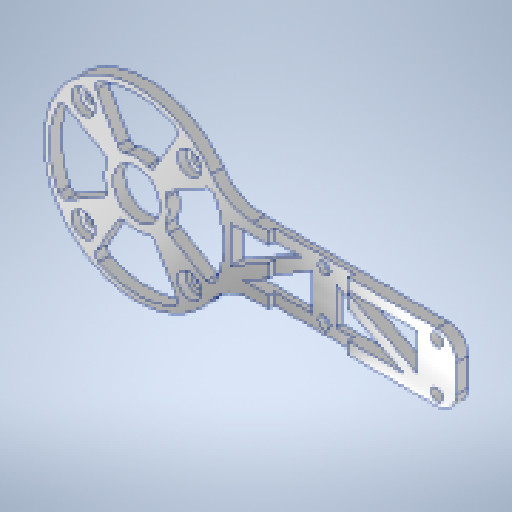
# Autodesk Inventor part: link2plate4
Saved by Autodesk Inventor 2024 (Build 280153000, 153)
## iProperties
Created: 2025-02-10
Part Number: link2plate4
Material: アルミニウム 6061
Document SubType Name: Modeling
Designer: tanoue_kota
Mass: 10.4195 g
Surface Area: 51.6889 cm^2
Volume: 3.85907 cm^3
Density: 2.7 g/cm^3
Appearance: アルミニウム - フラット
Author: tanoue_kota
Autodesk Inventor part; units mm, degrees
ref_plane "YZ Plane" through (0, 0, 0) normal (1, 0, 0) x (0, 1, 0)
ref_plane "XZ Plane" through (0, 0, 0) normal (0, 1, 0) x (-1, 0, 0)
ref_plane "XY Plane" through (0, 0, 0) normal (0, 0, 1) x (1, 0, 0)
sketch "スケッチ1" plane through (0, 0, 0) normal (0, 0, 1) x (1, 0, 0)
  line L0 (0, 0) -> (-81, 0)
  line L1 (-81, 0) -> (-81, 17)
  line L2 (-81, 17) -> (0, 17)
  line L3 (0, 17) -> (0, 0)
  line L4 (-81, 8.5) -> (0, 8.5)
  circle A0 centre (-81, 8.5) radius 23.5
  point P0 (-59.0911, 17)
  point P1 (-59.0911, 0)
  dimension "d0" = 17
  dimension "d28" = 47
  dimension "d29" = 81
  constraints: 10 end point, 2 midpoint, 2 parallel, 1 centre point, 1 coincident, 1 horizontal, 1 perpendicular
  measures "d0" distance of L2.end L0.start
  measures "d28" diameter of A0
  measures "d29" distance between parallel lines of L3 L1
extrude "押し出し1" add sketch "スケッチ1" along normal blind 3
sketch "スケッチ2" plane through (0, 0, 3) normal (0, 0, 1) x (1, 0, 0)
  line L0 (0, 0) -> (0, 17) projected
  line L1 (0, 8.5) -> (-59.0911, 8.5)
  line L2 (0, 17) -> (-59.0911, 17) projected
  line L3 (-5, 17) -> (-5, 0)
  line L4 (-35, 17) -> (-35, 0)
  line L5 (-59.0911, 0) -> (0, 0) projected
  arc A0 (-59.0911, 17) -> (-59.0911, 0) centre (-81, 8.5) ccw projected
  line L6 (-59.0911, 17) -> (-59.0911, 0)
  point P0 (-5, 14.5)
  point P1 (-35, 14.5)
  point P2 (-5, 2.5)
  point P3 (-35, 2.5)
  dimension "d4" = 5
  dimension "d5" = 30
  dimension "d6" = 6
  dimension "d7" = 6
  constraints: 8 end point, 5 point on line, 3 vertical, 2 midpoint, 2 symmetric about line, 1 parallel
  measures "d4" distance between parallel lines of L0 L3
  measures "d5" distance between parallel lines of L3 L4
  measures "d6" distance from line of L1 point (-5, 14.5)
  measures "d7" distance from line of L1 point (-35, 14.5)
hole "穴1" at (-5, 14.5, 3) at (-35, 14.5, 3) at (-35, 2.5, 3) at (-5, 2.5, 3) direction (0, 0, -1) diameter 3.1 depth 20 tip angle 118
sketch "スケッチ5" plane through (0, 0, 3) normal (0, 0, 1) x (1, 0, 0)
  arc A0 (-59.0911, 17) -> (-59.0911, 0) centre (-81, 8.5) ccw projected
  line L0 (-59.0911, 0) -> (0, 0) projected
  line L1 (0, 0) -> (0, 17) projected
  circle A1 centre (-81, 8.5) radius 19
  line L2 (-81, 8.5) -> (-81, 27.5)
  line L3 (-81, 8.5) -> (-94.435, 21.935)
  point P0 (-94.435, -4.935)
  point P1 (-67.565, -4.935)
  point P2 (-67.565, 21.935)
  dimension "d80" = 38
  dimension "d81" = 45
  dimension "d84" = 360
  constraints: 4 end point, 2 coincident, 2 point on circle, 1 centre point, 1 vertical, 5 other
  measures "d80" diameter of A1
  measures "d81" angle of L2 L3
hole "穴3" at (-67.565, 21.935, 3) at (-67.565, -4.935, 3) at (-94.435, -4.935, 3) at (-94.435, 21.935, 3) direction (0, 0, -1) diameter 3.1 end through all
sketch "スケッチ6" plane through (0, 0, 3) normal (0, 0, 1) x (1, 0, 0)
  arc A0 (-59.0911, 17) -> (-59.0911, 0) centre (-81, 8.5) ccw projected
  circle A1 centre (-81, 8.5) radius 6
  point P0 (0, 0)
  dimension "d43" = 12
  constraints: 1 centre point, 1 coincident
  measures "d43" diameter of A1
extrude "押し出し3" cut sketch "スケッチ6" against normal blind 3
sketch "スケッチ7" plane through (0, 0, 3) normal (0, 0, 1) x (1, 0, 0)
  circle A0 centre (-94.435, -4.935) radius 1.55 projected
  circle A1 centre (-67.565, -4.935) radius 1.55 projected
  circle A2 centre (-67.565, -4.935) radius 3
  circle A3 centre (-94.435, -4.935) radius 3
  circle A4 centre (-94.435, 21.935) radius 1.55 projected
  circle A5 centre (-94.435, 21.935) radius 3
  circle A6 centre (-67.565, 21.935) radius 1.55 projected
  circle A7 centre (-67.565, 21.935) radius 3
  point P0 (0, 0)
  dimension "d86" = 6
  dimension "d87" = 6
  dimension "d88" = 6
  dimension "d89" = 6
  constraints: 4 centre point, 4 coincident
  measures "d86" diameter of A2
  measures "d87" diameter of A3
  measures "d88" diameter of A5
  measures "d89" diameter of A7
extrude "押し出し4" cut sketch "スケッチ7" against normal blind 2 contours A0 | A1 | A2 | A3 | A4 | A5 | A6 | A7
sketch "スケッチ8" plane through (0, 0, 3) normal (0, 0, 1) x (1, 0, 0)
  line L0 (-81, 8.5) -> (-81, 30.5)
  line L1 (-81, 8.5) -> (-20.8346, 112.7096)
  line L2 (-77, 15.4282) -> (-20.8346, 112.7096)
  circle A0 centre (-81, 8.5) radius 22
  circle A1 centre (-81, 8.5) radius 8
  line L3 (0, 17) -> (-59.0911, 17) projected
  line L4 (-57, 17) -> (-57, -1.5)
  line L5 (-38, 17) -> (-38, 0)
  line L6 (-59.0911, 0) -> (0, 0) projected
  line L7 (-32, 17) -> (-32, 0)
  circle A2 centre (-35, 14.5) radius 1.55 projected
  line L8 (-10, 17) -> (-10, 0)
  line L9 (0, 0) -> (0, 17) projected
  line L10 (-57, 3) -> (0, 3)
  line L11 (-57, 14) -> (0, 14)
  line L12 (-57, 3) -> (-38, 14)
  line L13 (-57, 4.7332) -> (-40.9938, 14)
  line L14 (-54.0062, 3) -> (-38, 12.2668)
  line L15 (-32, 14) -> (-10, 3)
  line L16 (-32, 12.3229) -> (-13.3541, 3)
  line L17 (-28.6459, 14) -> (-10, 4.6771)
  line L18 (-85, 15.4282) -> (-141.1654, 112.7096)
  line L19 (-87.9282, 4.5) -> (-185.2096, -51.6654)
  line L20 (-81, 8.5) -> (-185.2096, 68.6654)
  line L21 (-77, 1.5718) -> (-20.8346, -95.7096)
  line L22 (-81, 8.5) -> (-141.1654, -95.7096)
  line L23 (-74.0718, 12.5) -> (23.2096, 68.6654)
  line L24 (-81, 8.5) -> (23.2096, -51.6654)
  circle A3 centre (-81, 8.5) radius 6 projected
  point P0 (-10, 14)
  point P1 (-32, 3)
  point P2 (-38, 3)
  point P3 (-87.9282, 12.5)
  point P4 (-85, 1.5718)
  point P5 (-74.0718, 4.5)
  point P6 (-85, 1.5718)
  point P7 (-92, -10.5526)
  point P8 (-70, -10.5526)
  point P9 (-77, 1.5718)
  point P10 (-74.0718, 4.5)
  point P11 (-61.9474, -2.5)
  point P12 (-61.9474, 19.5)
  point P13 (-74.0718, 12.5)
  point P14 (-92, 27.5526)
  point P15 (-85, 15.4282)
  point P16 (-70, 27.5526)
  point P17 (-87.9282, 12.5)
  point P18 (-100.0526, 19.5)
  point P19 (-100.0526, -2.5)
  point P20 (-87.9282, 4.5)
  dimension "d57" = 44
  dimension "d69" = 16
  dimension "d52" = 30
  dimension "d58" = 24
  dimension "d59" = 3
  dimension "d60" = 3
  dimension "d61" = 10
  dimension "d62" = 3
  dimension "d63" = 3
  dimension "d64" = 1.5
  dimension "d66" = 1.5
  dimension "d67" = 1.5
  dimension "d68" = 1.5
  dimension "d74" = 360
  constraints: 44 end point, 26 point on line, 5 coincident, 5 parallel, 4 vertical, 2 perpendicular, 2 symmetric about line, 1 collinear, 38 other
  measures "d52" angle of L0 L1
  measures "d58" distance from line of point (-81, 8.5) L4
  measures "d59" distance from line of L5 A2.centre
  measures "d60" distance from line of A2.centre L7
  measures "d61" distance between parallel lines of L9 L8
  measures "d62" distance between parallel lines of L3 L11
  measures "d63" distance of the line from the sketch origin of L10
  measures "d64" distance between parallel lines of L12 L13
  measures "d66" distance between parallel lines of L12 L14
  measures "d67" distance between parallel lines of L15 L17
  measures "d68" distance between parallel lines of L15 L16
extrude "押し出し5" cut sketch "スケッチ8" against normal blind 3 contours A1 L18 A0 L0 | L0 A0 L1 A1 | A1 L19 A0 L20 | A1 L21 A0 L22 | A1 L23 A0 L24 | L8 L17 L11 | L16 L10 L7 | L11 L13 L4 | L5 L10 L14
fillet "フィレット1" radius 1.5 16 edges at (-100.0526, 19.5, 1.5) (-87.9282, 12.5, 1.5) (-85, 15.4282, 1.5) (-92, 27.5526, 1.5) (-70, 27.5526, 1.5) (-77, 15.4282, 1.5) (-74.0718, 12.5, 1.5) (-61.9474, 19.5, 1.5) (-74.0718, 4.5, 1.5) (-61.9474, -2.5, 1.5) (-70, -10.5526, 1.5) (-77, 1.5718, 1.5) (-85, 1.5718, 1.5) (-92, -10.5526, 1.5) (-87.9282, 4.5, 1.5) (-100.0526, -2.5, 1.5)
fillet "フィレット2" radius 13 2 edges at (-59.0911, 17, 1.5) (-59.0911, 0, 1.5)
fillet "フィレット3" radius 5 2 edges at (0, 17, 1.5) (0, 0, 1.5)
sketch "スケッチ9" plane through (0, 0, 3) normal (0, 0, 1) x (1, 0, 0)
  line L0 (-51.5042, 0) -> (-5, 0) projected
  line L1 (-27.5, 0) -> (-27.5, 17)
  line L2 (-5, 17) -> (-51.5042, 17) projected
  line L3 (-47.5, 0) -> (-47.5, 17)
  line L4 (0, 5) -> (0, 12) projected
  point P0 (0, 0)
  point P1 (-47.5, 17)
  point P2 (-47.5, 0)
  dimension "d90" = 27.5
  dimension "d91" = 20
  constraints: 4 end point, 2 point on line, 2 vertical
  measures "d90" distance between parallel lines of L4 L1
  measures "d91" distance between parallel lines of L1 L3
extrude "押し出し6" cut sketch "スケッチ9" against normal blind 1.5
